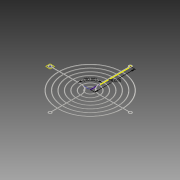
# Autodesk Inventor part: Grill
Saved by Autodesk Inventor 2016 (Build 200138000, 138)
## iProperties
Created: 2015-10-19
Part Number: Grill
Material: Generic
Document SubType Name: Modeling
Designer: Rus
Density: 1 g/cm^3
Appearance: Default
Author: Rus
Autodesk Inventor part; units mm, degrees
ref_plane "YZ Plane" through (0, 0, 0) normal (1, 0, 0) x (0, 1, 0)
ref_plane "XZ Plane" through (0, 0, 0) normal (0, 1, 0) x (-1, 0, 0)
ref_plane "XY Plane" through (0, 0, 0) normal (0, 0, 1) x (1, 0, 0)
sketch "Sketch1" plane through (0, 0, 0) normal (0, 0, 1) x (1, 0, 0)
  line L0 (0, 98.9949) -> (98.9949, 0)
  line L1 (98.9949, 0) -> (0, -98.9949)
  line L2 (0, -98.9949) -> (-98.9949, 0)
  line L3 (-98.9949, 0) -> (0, 98.9949)
  line L4 (0, 98.9949) -> (0, -98.9949) construction
  line L5 (98.9949, 0) -> (-98.9949, 0) construction
  line L6 (0, 98.9949) -> (140, 98.9949) construction
  line L7 (0, 0) -> (80, 0)
  line L8 (0, 0) -> (0, 80)
  line L9 (0, 0) -> (0, 10)
  line L10 (0, 10) -> (0, 20)
  line L11 (0, 20) -> (0, 30)
  line L12 (0, 30) -> (0, 40)
  line L13 (0, 40) -> (0, 50)
  line L14 (0, 50) -> (0, 60)
  line L15 (0, 60) -> (0, 70)
  line L16 (0, 70) -> (0, 80)
  dimension "d0" = 140
  dimension "d1" = 45
  dimension "d2" = 140
  dimension "d3" = 80
  dimension "d4" = 80
  dimension "d5" = 10
  dimension "d6" = 10
  dimension "d7" = 10
  dimension "d8" = 10
  dimension "d9" = 10
  dimension "d10" = 10
  dimension "d11" = 10
  dimension "d12" = 10
  constraints: 32 end point, 8 coincident, 4 equal length, 3 midpoint, 2 point on line, 1 horizontal, 1 perpendicular, 10 other
  measures "d0" distance of L0.start L0.end
  measures "d1" angle of L0 L6
  measures "d2" distance of L0.end L1.end
  measures "d3" distance of L7.start L7.end
  measures "d4" distance of L9.start L16.end
  measures "d5" distance of L9.start L9.end
  measures "d6" distance of L9.end L10.end
  measures "d7" distance of L10.end L11.end
  measures "d8" distance of L11.end L12.end
  measures "d9" distance of L12.end L13.end
  measures "d10" distance of L13.end L14.end
  measures "d11" distance of L14.end L15.end
  measures "d12" distance of L15.end L16.end
ref_plane "Work Plane1" through (-98.9949, 0, 0) normal (0, 0, -1) x (0.7071068, 0.7071068, 0)
sketch "Sketch2" plane through (0, 0, 0) normal (1, 0, 0) x (0, 1, 0)
  circle A0 centre (10, 0) radius 1
  circle A1 centre (20, 0) radius 1
  circle A2 centre (30, 0) radius 1
  circle A3 centre (40, 0) radius 1
  circle A4 centre (50, 0) radius 1
  circle A5 centre (60, 0) radius 1
  circle A6 centre (70, 0) radius 1
  circle A7 centre (80, 0) radius 1
  line L0 (0, 1.4) -> (0, -1.4) projected
  point P0 (0, 0)
  dimension "d13" = 2
  dimension "d14" = 2
  dimension "d15" = 2
  dimension "d16" = 2
  dimension "d17" = 2
  dimension "d18" = 2
  dimension "d19" = 2
  dimension "d20" = 2
  constraints: 8 centre point, 8 coincident
  measures "d13" diameter of A0
  measures "d14" diameter of A1
  measures "d15" diameter of A2
  measures "d16" diameter of A3
  measures "d17" diameter of A4
  measures "d18" diameter of A5
  measures "d19" diameter of A6
  measures "d20" diameter of A7
revolve "Revolution1" add sketch "Sketch2" angle 360 about axis through (0, 0, 0) along (0, 0, -1)
ref_plane "Work Plane2" through (0, 0, 0) normal (0, 0, -1) x (-1, 0, 0)
sketch "Sketch3" plane through (0, 0, 0) normal (0, 0, -1) x (-1, 0, 0)
  line L0 (0, 20) -> (0, 85.035)
  line L1 (-20, 0) -> (-85.035, 0)
  arc A0 (-20, 0) -> (0, 20) centre (-20, 20) ccw
  line L2 (20, 0) -> (85.035, 0)
  line L3 (0, -20) -> (0, -85.035)
  arc A1 (20, 0) -> (0, -20) centre (20, -20) ccw
  point P0 (0, 0)
  dimension "d22" = 85.035
  dimension "d23" = 85.035
  dimension "d24" = 20
  dimension "d25" = 85.035
  dimension "d26" = 85.035
  dimension "d27" = 20
  constraints: 8 end point, 4 point on circle, 4 point on line, 4 tangent, 2 centre point, 2 horizontal, 2 vertical
  measures "d22" distance of point (0, 0) L0.end
  measures "d23" distance of point (0, 0) L1.end
  measures "d24" radius of A0
  measures "d25" distance of point (0, 0) L2.end
  measures "d26" distance of point (0, 0) L3.end
  measures "d27" radius of A1
ref_plane "Work Plane3" through (-20, 0, 0) normal (0, -1, 0) x (-1, 0, 0)
ref_plane "Work Plane4" through (0, 0, 0) normal (-1, 0, 0) x (0, 0, -1)
ref_plane "Work Plane5" through (0, 85.035, 0) normal (0, -1, 0) x (-1, 0, 0)
sketch "Sketch4" plane through (0, 85.035, 0) normal (0, -1, 0) x (-1, 0, 0)
  circle A0 centre (0, -2) radius 1
  line L0 (80, -1) -> (-80, -1) projected
  point P0 (0, 0)
  point P1 (0, -1)
  dimension "d29" = 2
  constraints: 1 midpoint, 1 vertical alignment, 2 other
ref_plane "Work Plane6" through (0, -85.035, 0) normal (0, -1, 0) x (-1, 0, 0)
sketch "Sketch5" plane through (0, -85.035, 0) normal (0, -1, 0) x (-1, 0, 0)
  circle A0 centre (0, -2) radius 1
  point P0 (0, 0)
  point P1 (0, -2)
  dimension "d30" = 2
  constraints: 1 centre point, 1 coincident
  measures "d30" diameter of A0
sweep "Sweep1" add profiles "Sketch5" path "Sketch3" path curves L3 A1 L2
sweep "Sweep2" add profiles "Sketch4" path "Sketch3" path curves L0 A0 L1
sketch "Sketch6" plane through (0, 85.035, 2) normal (0, 1, 0) x (1, 0, 0)
  point P0 (0, 2)
  point P1 (0, 0)
ref_plane "Work Plane8" through (0, 85.035, 2) normal (0, 0, -1) x (-1, 0, 0)
ref_plane "Work Plane7" through (0, 0, 0) normal (0, 0, -1) x (-1, 0, 0)
sketch "Sketch7" plane through (0, 85.035, 2) normal (0, 0, -1) x (-1, 0, 0)
  line L0 (1, -105.035) -> (-1, -105.035) projected
  line L1 (1, -170.07) -> (-1, -170.07) projected
  line L2 (-1, -65.035) -> (1, -65.035) projected
  line L3 (1, 0) -> (-1, 0) projected
  line L4 (85.035, -86.035) -> (85.035, -84.035) projected
  line L5 (20, -86.035) -> (20, -84.035) projected
  line L6 (-85.035, -84.035) -> (-85.035, -86.035) projected
  line L7 (-20, -84.035) -> (-20, -86.035) projected
  circle A0 centre (0, -173.07) radius 3
  line L8 (1, -170.07) -> (-1, -170.07) projected
  circle A1 centre (88.035, -85.035) radius 3
  circle A2 centre (0, 3) radius 3
  circle A3 centre (-88.035, -85.035) radius 3
  point P0 (0, -85.035)
  point P1 (0, -155.035)
  point P2 (0, -135.035)
  point P3 (0, -125.035)
  point P4 (0, -165.035)
  point P5 (0, -105.035)
  point P6 (0, -5.035)
  point P7 (0, -45.035)
  point P8 (0, -35.035)
  point P9 (0, -15.035)
  point P10 (0, -65.035)
  point P11 (70, -85.035)
  point P12 (50, -85.035)
  point P13 (40, -85.035)
  point P14 (80, -85.035)
  point P15 (20, -85.035)
  point P16 (-80, -85.035)
  point P17 (-40, -85.035)
  point P18 (-50, -85.035)
  point P19 (-70, -85.035)
  point P20 (-20, -85.035)
  point P21 (0, -170.07)
  point P22 (85.035, -85.035)
  point P23 (0, 0)
  point P24 (-85.035, -85.035)
  dimension "d35" = 6
  dimension "d38" = 360
  constraints: 2 horizontal alignment, 2 vertical alignment, 1 horizontal, 1 midpoint, 21 other
ref_plane "Work Plane9" through (0, 85.035, 2) normal (1, 0, 0) x (0, 1, 0)
sketch "Sketch8" plane through (0, 85.035, 2) normal (1, 0, 0) x (0, 1, 0)
  circle A0 centre (0, 0) radius 1
  point P0 (-85.035, -2)
  dimension "d40" = 2
  constraints: 1 centre point
  measures "d40" diameter of A0
sketch "Sketch9" plane through (0, 85.035, 2) normal (1, 0, 0) x (0, 1, 0)
  line L0 (-170.07, -1) -> (-170.07, 1) projected
  circle A0 centre (-170.07, 0) radius 1
  point P0 (-85.035, -2)
  dimension "d41" = 2
  constraints: 1 centre point, 1 midpoint
  measures "d41" diameter of A0
ref_plane "Work Plane10" through (85.035, 0, 2) normal (0, 1, 0) x (1, 0, 0)
sketch "Sketch10" plane through (85.035, 0, 2) normal (0, 1, 0) x (1, 0, 0)
  line L0 (0, -1) -> (0, 1) projected
  circle A0 centre (0, 0) radius 1
  line L1 (-170.07, 1) -> (-170.07, -1) projected
  circle A1 centre (-170.07, 0) radius 1
  point P0 (-85.035, 2)
  dimension "d42" = 2
  dimension "d43" = 2
  constraints: 2 centre point, 2 midpoint
  measures "d42" diameter of A0
  measures "d43" diameter of A1
sweep "Sweep3" add profiles "Sketch10" path "Sketch7" path curves A3 contours A0 L0 | L0 A0
sweep "Sweep4" add profiles "Sketch8" path "Sketch7" path curves A2
sweep "Sweep5" add profiles "Sketch10" path "Sketch7" path curves A1 contours A1 L1 | L1 A1
sweep "Sweep6" add profiles "Sketch9" path "Sketch7" path curves A0
ref_plane "Work Plane11" through (85.035, 0, 1) normal (0, 0, -1) x (-1, 0, 0)
sketch "Sketch11" plane through (85.035, 0, 1) normal (0, 0, -1) x (-1, 0, 0)
  circle A0 centre (85.035, 0) radius 75.1001
  circle A1 centre (85.035, 0) radius 119.8876
  constraints: 2 centre point, 2 coincident
extrude "Extrusion1" cut sketch "Sketch11" along normal blind 10
ref_plane "Work Plane12" through (-88.035, 0, 2) normal (0, 0, -1) x (-1, 0, 0)
sketch "Sketch12" plane through (-88.035, 0, 2) normal (0, 0, -1) x (-1, 0, 0)
  line L0 (-88.035, 0) -> (-88.035, 88.035)
  line L1 (-89.035, 84.162) -> (-89.035, 20) projected
  line L2 (-88.035, 0) -> (0, 0) construction
  circle A0 centre (-88.035, 88.035) radius 2 projected
  line L3 (-88.035, 88.035) -> (-88.035, 88.035)
  dimension "d54" = 88.035
  dimension "d55" = 90
  constraints: 6 end point, 1 collinear, 1 horizontal, 1 parallel, 1 perpendicular
  measures "d54" distance of L0.start L0.end
  measures "d55" angle of L2 L0
body "Solid1"
